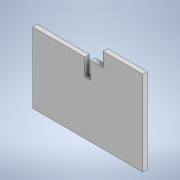
# Autodesk Inventor part: pcb_balun_bottom
Saved by Autodesk Inventor 2020.2 (Build 242310000, 310)
## iProperties
Created: 2020-09-26
Part Number: pcb_balun_bottom
Material: Generic
Document SubType Name: Modeling
Designer: Krishna Makhija
Density: 1 g/cm^3
Appearance: Default
Author: Krishna Makhija
Autodesk Inventor part; units mm, degrees
ref_plane "YZ Plane" through (0, 0, 0) normal (1, 0, 0) x (0, 1, 0)
ref_plane "XZ Plane" through (0, 0, 0) normal (0, 1, 0) x (-1, 0, 0)
ref_plane "XY Plane" through (0, 0, 0) normal (0, 0, 1) x (1, 0, 0)
sketch "Sketch4" plane through (0, 0, 0) normal (0, 0, 1) x (1, 0, 0)
  line L0 (19.5002, -12.5002) -> (-19.5002, -12.5002)
  line L1 (-19.5002, -12.5002) -> (-19.5002, 12.5002)
  line L2 (19.5002, 12.5002) -> (19.5002, -12.5002)
  line L3 (19.5002, -12.5002) -> (-19.5002, 12.5002) construction
  line L4 (-19.5002, -12.5002) -> (19.5002, 12.5002) construction
  line L5 (5.5006, 12.5002) -> (5.5006, 17.5003)
  line L6 (5.5006, 17.5003) -> (19.5002, 17.5003)
  line L7 (19.5002, 17.5003) -> (19.5002, 12.5002)
  line L8 (0.9999, 6.5006) -> (-0.9999, 6.5006)
  line L9 (-0.9999, 6.5006) -> (-0.9999, 12.5002)
  line L10 (0.9999, 12.5002) -> (0.9999, 6.5006)
  line L11 (0.9999, 6.5006) -> (-0.9999, 12.5002) construction
  line L12 (-0.9999, 6.5006) -> (0.9999, 12.5002) construction
  line L13 (-0.9999, 12.5002) -> (-19.5002, 12.5002)
  line L14 (0.9999, 12.5002) -> (5.5006, 12.5002)
  constraints: 30 end point, 3 horizontal, 3 parallel, 2 perpendicular, 1 collinear
extrude "Extrusion3" add sketch "Sketch4" along normal blind 1.6
body "Solid3"
